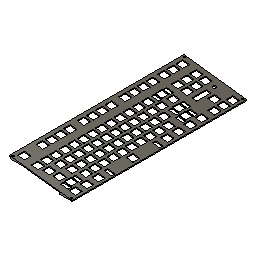
case-top (Autodesk Fusion 360 design; units mm, degrees)
part number: 2025-12-05-19-02-36-904
Autodesk Fusion 360 part; units mm, degrees
(part 1 of 2)
sketch "middle-side-profile" plane through (0, 0, 0) normal (0, 1, 0) x (1, 0, 0)
  line L0 (-127.2538, 3.7478) -> (-128.8538, 3.7478)
  line L1 (-128.8538, -15.8213) -> (-126.4008, -15.5201)
  line L2 (-126.4008, -15.5201) -> (-127.0101, -10.5573)
  line L3 (-128.8538, 3.7478) -> (-128.8538, -15.8213)
  line L4 (-127.0101, -10.5573) -> (-10.504, 3.7478)
  line L5 (-10.504, 3.7478) -> (-56.2538, 3.7478)
  line L6 (0, 0) -> (-128.8538, -15.8213)
  line L7 (-128.8538, 3.7478) -> (0, 3.7478)
  line L8 (0, 3.7478) -> (0, 0)
  line L9 (-24.433, 3.7478) -> (-24.433, -3)
  line L10 (0, 0) -> (-24.433, 0)
  line L11 (-126.3318, -16.082) -> (-126.9165, -11.3197)
  line L12 (-126.7691, -12.5201) -> (-101.9677, -12.5201)
  line L13 (0, 0) -> (0.2437, -1.9851)
  line L14 (-128.8538, -15.8213) -> (-128.6101, -17.8064)
  line L15 (-128.6101, -17.8064) -> (0.2437, -1.9851)
  line L16 (0, 3.7478) -> (1.6, 3.7478)
  line L17 (0.2437, -1.9851) -> (1.6, -1.8186)
  line L18 (1.6, -1.8186) -> (1.6, 3.7478)
  line L19 (0, 0) -> (1.6, 0.1965)
  line L20 (0, 0) -> (1.612, 0) construction
  dimension "d1" = 2
  dimension "d2" = 2
  dimension "d7" = 1.6
  dimension "d8" = 7
  constraint coincident L6.start L8.end
  constraint perpendicular L6 L13
  constraint perpendicular L6 L14
  constraint perpendicular L13 L15
  constraint perpendicular L8 L16
  constraint perpendicular L13 L17
  constraint perpendicular L16 L18
  constraint horizontal L20
  constraint coincident L18 L19.end
  measures "d1" distance of L6.start L13.end
  measures "d2" distance of L1.start L14.end
  measures "d7" distance of L7.end L16.end
  measures "d8" angle of L19 L20
extrude "Extrude1" add sketch "middle-side-profile" along normal blind 362.2 contours L1 L6 L13 L14 L15 | L2 L6 L11 L12 | L13 L17 L18 L19 | L6 L9 L10
sketch "Sketch2" plane through (0, 0, 0) normal (0, 0, -1) x (1, 0, 0)
  line L0 (0, 0) -> (-24.433, 0)
  line L1 (-24.433, 0) -> (-24.433, -362.2)
  line L2 (-24.433, -362.2) -> (0, -362.2)
  line L3 (0, 0) -> (-128.854, 0)
  line L4 (-128.854, 0) -> (-128.854, -362.2)
  line L5 (-128.854, -362.2) -> (0, -362.2)
  line L6 (0, -362.2) -> (0, 0)
  line L7 (0, -362.2) -> (0, 0)
  line L8 (0, -181.1) -> (-128.854, -181.1)
  circle A0 centre (-3.2, -3.2) radius 1.55
  line L9 (1.6, 0) -> (1.6, -362.2)
  circle A1 centre (-124.054, -3.2) radius 1.55
  circle A2 centre (-3.2, -359) radius 1.55
  circle A3 centre (-124.054, -359) radius 1.55
  dimension "d5" = 128.854
  dimension "d6" = 362.2
  dimension "d11" = 181.1
  dimension "d12" = 3.1
  dimension "d13" = 4.8
  dimension "d14" = 3.2
  dimension "d15" = 3.1
  dimension "d16" = 3.2
  dimension "d17" = 4.8
  dimension "d18" = 3.1
  dimension "d19" = 3.2
  dimension "d20" = 4.8
  dimension "d21" = 3.1
  dimension "d22" = 4.8
  dimension "d23" = 3.2
  constraint horizontal L3
  constraint vertical L4
  constraint horizontal L5
  constraint vertical L6
  constraint coincident L0.start L3.start
  constraint coincident L7 L8.start
  constraint coincident L4 L8.end
  constraint perpendicular L4 L8
  measures "d5" distance of L0.start L3.end
  measures "d6" distance of L0.start L2.end
  measures "d11" distance of L5 L8
  measures "d12" diameter of A0
  measures "d13" distance of A0.centre L9
  measures "d14" distance of L3 A0.centre
  measures "d15" diameter of A1
  measures "d16" distance of L3 A1.centre
  measures "d17" distance of L4 A1.centre
  measures "d18" diameter of A2
  measures "d19" distance of L5 A2.centre
  measures "d20" distance of L9 A2.centre
  measures "d21" diameter of A3
  measures "d22" distance of L4 A3.centre
  measures "d23" distance of L5 A3.centre
hole "Hole1" at (-124.054, 359, 0) direction (0, 0, 1) diameter 2.2 depth 15 tip angle 180
hole "Hole2" at (-3.2, 359, 0) direction (0, 0, 1) diameter 2.2 depth 1 tip angle 180
hole "Hole3" at (-3.2, 3.2, 0) direction (0, 0, 1) diameter 2.2 depth 1 tip angle 180
hole "Hole4" at (-124.054, 3.2, 0) direction (0, 0, 1) diameter 2.2 depth 15 tip angle 180
ref_plane "WorkPlane1" through (0, 0, 20) normal (0, 0, 1) x (1, 0, 0)
sketch "Sketch4" plane through (0, 0, 20) normal (0, 0, 1) x (1, 0, 0)
  line L0 (1.6, 0) -> (-128.854, 0)
  line L1 (-128.854, 0) -> (-128.854, -362.2)
  line L2 (-128.854, -362.2) -> (1.6, -362.2)
  line L3 (1.6, -362.2) -> (1.6, 0)
  circle A0 centre (-124.0538, 3.2) radius 2
  line L4 (-128.8538, 0) -> (-128.8538, 362.2)
  circle A1 centre (-124.0538, 359) radius 2
  line L5 (-128.6101, 362.2) -> (1.6, 362.2)
  circle A2 centre (-3.2, 359) radius 2
  line L6 (1.6, 0) -> (1.6, 362.2)
  circle A3 centre (-3.2, 3.2) radius 2
  dimension "d46" = 130.454
  dimension "d47" = 362.2
  dimension "d48" = 4
  dimension "d49" = 4.8
  dimension "d50" = 3.2
  dimension "d51" = 4
  dimension "d52" = 4.8
  dimension "d53" = 3.2
  dimension "d54" = 4
  dimension "d55" = 4.8
  dimension "d56" = 3.2
  dimension "d57" = 4
  dimension "d58" = 3.2
  dimension "d59" = 4.8
  constraint horizontal L0
  constraint vertical L1
  constraint horizontal L2
  constraint vertical L3
  measures "d46" distance of L0.start L0.end
  measures "d47" distance of L0.start L2.end
  measures "d48" diameter of A0
  measures "d49" distance of A0.centre L4
  measures "d50" distance of L0 A0.centre
  measures "d51" diameter of A1
  measures "d52" distance of L4 A1.centre
  measures "d53" distance of A1.centre L5
  measures "d54" diameter of A2
  measures "d55" distance of A2.centre L6
  measures "d56" distance of L5 A2.centre
  measures "d57" diameter of A3
  measures "d58" distance of L0 A3.centre
  measures "d59" distance of L6 A3.centre
hole "Hole6" at (-124.0538, 3.2, 20) direction (0, 0, -1) diameter 4 depth 5 tip angle 180
hole "Hole7" at (-3.2, 3.2, 20) direction (0, 0, -1) diameter 4 depth 19 tip angle 180
hole "Hole8" at (-3.2, 359, 20) direction (0, 0, -1) diameter 4 depth 19 tip angle 180
hole "Hole9" at (-124.0538, 359, 20) direction (0, 0, -1) diameter 4 depth 19 tip angle 180
sketch "plate-2025-12-06T02_04_04.924Z" plane through (0.2437, 0, 1.9851) normal (0.121869, 0, 0.992546) x (0.992546, 0, -0.121869)
  line L0 (-122.5865, 10.3145) -> (-122.5865, 23.3145)
  line L1 (-108.5865, 10.3145) -> (-108.5865, 23.3145)
  line L2 (-122.0865, 9.8145) -> (-109.0865, 9.8145)
  line L3 (-122.0865, 23.8145) -> (-109.0865, 23.8145)
  arc A0 (-122.5865, 10.3145) -> (-122.0865, 9.8145) centre (-122.0865, 10.3145) ccw
  arc A1 (-122.0865, 23.8145) -> (-122.5865, 23.3145) centre (-122.0865, 23.3145) ccw
  arc A2 (-109.0865, 9.8145) -> (-108.5865, 10.3145) centre (-109.0865, 10.3145) ccw
  arc A3 (-108.5865, 23.3145) -> (-109.0865, 23.8145) centre (-109.0865, 23.3145) ccw
  line L4 (-122.5865, 48.4145) -> (-122.5865, 61.4145)
  line L5 (-108.5865, 48.4145) -> (-108.5865, 61.4145)
  line L6 (-122.0865, 47.9145) -> (-109.0865, 47.9145)
  line L7 (-122.0865, 61.9145) -> (-109.0865, 61.9145)
  arc A4 (-122.5865, 48.4145) -> (-122.0865, 47.9145) centre (-122.0865, 48.4145) ccw
  arc A5 (-122.0865, 61.9145) -> (-122.5865, 61.4145) centre (-122.0865, 61.4145) ccw
  arc A6 (-109.0865, 47.9145) -> (-108.5865, 48.4145) centre (-109.0865, 48.4145) ccw
  arc A7 (-108.5865, 61.4145) -> (-109.0865, 61.9145) centre (-109.0865, 61.4145) ccw
  line L8 (-122.5865, 67.4645) -> (-122.5865, 80.4645)
  line L9 (-108.5865, 67.4645) -> (-108.5865, 80.4645)
  line L10 (-122.0865, 66.9645) -> (-109.0865, 66.9645)
  line L11 (-122.0865, 80.9645) -> (-109.0865, 80.9645)
  arc A8 (-122.5865, 67.4645) -> (-122.0865, 66.9645) centre (-122.0865, 67.4645) ccw
  arc A9 (-122.0865, 80.9645) -> (-122.5865, 80.4645) centre (-122.0865, 80.4645) ccw
  arc A10 (-109.0865, 66.9645) -> (-108.5865, 67.4645) centre (-109.0865, 67.4645) ccw
  arc A11 (-108.5865, 80.4645) -> (-109.0865, 80.9645) centre (-109.0865, 80.4645) ccw
  line L12 (-122.5865, 86.5145) -> (-122.5865, 99.5145)
  line L13 (-108.5865, 86.5145) -> (-108.5865, 99.5145)
  line L14 (-122.0865, 86.0145) -> (-109.0865, 86.0145)
  line L15 (-122.0865, 100.0145) -> (-109.0865, 100.0145)
  arc A12 (-122.5865, 86.5145) -> (-122.0865, 86.0145) centre (-122.0865, 86.5145) ccw
  arc A13 (-122.0865, 100.0145) -> (-122.5865, 99.5145) centre (-122.0865, 99.5145) ccw
  arc A14 (-109.0865, 86.0145) -> (-108.5865, 86.5145) centre (-109.0865, 86.5145) ccw
  arc A15 (-108.5865, 99.5145) -> (-109.0865, 100.0145) centre (-109.0865, 99.5145) ccw
  line L16 (-122.5865, 105.5645) -> (-122.5865, 118.5645)
  line L17 (-108.5865, 105.5645) -> (-108.5865, 118.5645)
  line L18 (-122.0865, 105.0645) -> (-109.0865, 105.0645)
  line L19 (-122.0865, 119.0645) -> (-109.0865, 119.0645)
  arc A16 (-122.5865, 105.5645) -> (-122.0865, 105.0645) centre (-122.0865, 105.5645) ccw
  arc A17 (-122.0865, 119.0645) -> (-122.5865, 118.5645) centre (-122.0865, 118.5645) ccw
  arc A18 (-109.0865, 105.0645) -> (-108.5865, 105.5645) centre (-109.0865, 105.5645) ccw
  arc A19 (-108.5865, 118.5645) -> (-109.0865, 119.0645) centre (-109.0865, 118.5645) ccw
  line L20 (-122.5865, 134.1395) -> (-122.5865, 147.1395)
  line L21 (-108.5865, 134.1395) -> (-108.5865, 147.1395)
  line L22 (-122.0865, 133.6395) -> (-109.0865, 133.6395)
  line L23 (-122.0865, 147.6395) -> (-109.0865, 147.6395)
  arc A20 (-122.5865, 134.1395) -> (-122.0865, 133.6395) centre (-122.0865, 134.1395) ccw
  arc A21 (-122.0865, 147.6395) -> (-122.5865, 147.1395) centre (-122.0865, 147.1395) ccw
  arc A22 (-109.0865, 133.6395) -> (-108.5865, 134.1395) centre (-109.0865, 134.1395) ccw
  arc A23 (-108.5865, 147.1395) -> (-109.0865, 147.6395) centre (-109.0865, 147.1395) ccw
  line L24 (-122.5865, 153.1895) -> (-122.5865, 166.1895)
  line L25 (-108.5865, 153.1895) -> (-108.5865, 166.1895)
  line L26 (-122.0865, 152.6895) -> (-109.0865, 152.6895)
  line L27 (-122.0865, 166.6895) -> (-109.0865, 166.6895)
  arc A24 (-122.5865, 153.1895) -> (-122.0865, 152.6895) centre (-122.0865, 153.1895) ccw
  arc A25 (-122.0865, 166.6895) -> (-122.5865, 166.1895) centre (-122.0865, 166.1895) ccw
  arc A26 (-109.0865, 152.6895) -> (-108.5865, 153.1895) centre (-109.0865, 153.1895) ccw
  arc A27 (-108.5865, 166.1895) -> (-109.0865, 166.6895) centre (-109.0865, 166.1895) ccw
  line L28 (-122.5865, 172.2395) -> (-122.5865, 185.2395)
  line L29 (-108.5865, 172.2395) -> (-108.5865, 185.2395)
  line L30 (-122.0865, 171.7395) -> (-109.0865, 171.7395)
  line L31 (-122.0865, 185.7395) -> (-109.0865, 185.7395)
  arc A28 (-122.5865, 172.2395) -> (-122.0865, 171.7395) centre (-122.0865, 172.2395) ccw
  arc A29 (-122.0865, 185.7395) -> (-122.5865, 185.2395) centre (-122.0865, 185.2395) ccw
  arc A30 (-109.0865, 171.7395) -> (-108.5865, 172.2395) centre (-109.0865, 172.2395) ccw
  arc A31 (-108.5865, 185.2395) -> (-109.0865, 185.7395) centre (-109.0865, 185.2395) ccw
  line L32 (-122.5865, 191.2895) -> (-122.5865, 204.2895)
  line L33 (-108.5865, 191.2895) -> (-108.5865, 204.2895)
  line L34 (-122.0865, 190.7895) -> (-109.0865, 190.7895)
  line L35 (-122.0865, 204.7895) -> (-109.0865, 204.7895)
  arc A32 (-122.5865, 191.2895) -> (-122.0865, 190.7895) centre (-122.0865, 191.2895) ccw
  arc A33 (-122.0865, 204.7895) -> (-122.5865, 204.2895) centre (-122.0865, 204.2895) ccw
  arc A34 (-109.0865, 190.7895) -> (-108.5865, 191.2895) centre (-109.0865, 191.2895) ccw
  arc A35 (-108.5865, 204.2895) -> (-109.0865, 204.7895) centre (-109.0865, 204.2895) ccw
  line L36 (-122.5865, 219.8645) -> (-122.5865, 232.8645)
  line L37 (-108.5865, 219.8645) -> (-108.5865, 232.8645)
  line L38 (-122.0865, 219.3645) -> (-109.0865, 219.3645)
  line L39 (-122.0865, 233.3645) -> (-109.0865, 233.3645)
  arc A36 (-122.5865, 219.8645) -> (-122.0865, 219.3645) centre (-122.0865, 219.8645) ccw
  arc A37 (-122.0865, 233.3645) -> (-122.5865, 232.8645) centre (-122.0865, 232.8645) ccw
  arc A38 (-109.0865, 219.3645) -> (-108.5865, 219.8645) centre (-109.0865, 219.8645) ccw
  arc A39 (-108.5865, 232.8645) -> (-109.0865, 233.3645) centre (-109.0865, 232.8645) ccw
  line L40 (-122.5865, 238.9145) -> (-122.5865, 251.9145)
  line L41 (-108.5865, 238.9145) -> (-108.5865, 251.9145)
  line L42 (-122.0865, 238.4145) -> (-109.0865, 238.4145)
  line L43 (-122.0865, 252.4145) -> (-109.0865, 252.4145)
  arc A40 (-122.5865, 238.9145) -> (-122.0865, 238.4145) centre (-122.0865, 238.9145) ccw
  arc A41 (-122.0865, 252.4145) -> (-122.5865, 251.9145) centre (-122.0865, 251.9145) ccw
  arc A42 (-109.0865, 238.4145) -> (-108.5865, 238.9145) centre (-109.0865, 238.9145) ccw
  arc A43 (-108.5865, 251.9145) -> (-109.0865, 252.4145) centre (-109.0865, 251.9145) ccw
  line L44 (-122.5865, 257.9645) -> (-122.5865, 270.9645)
  line L45 (-108.5865, 257.9645) -> (-108.5865, 270.9645)
  line L46 (-122.0865, 257.4645) -> (-109.0865, 257.4645)
  line L47 (-122.0865, 271.4645) -> (-109.0865, 271.4645)
  arc A44 (-122.5865, 257.9645) -> (-122.0865, 257.4645) centre (-122.0865, 257.9645) ccw
  arc A45 (-122.0865, 271.4645) -> (-122.5865, 270.9645) centre (-122.0865, 270.9645) ccw
  arc A46 (-109.0865, 257.4645) -> (-108.5865, 257.9645) centre (-109.0865, 257.9645) ccw
  arc A47 (-108.5865, 270.9645) -> (-109.0865, 271.4645) centre (-109.0865, 270.9645) ccw
  line L48 (-122.5865, 277.0145) -> (-122.5865, 290.0145)
  line L49 (-108.5865, 277.0145) -> (-108.5865, 290.0145)
  line L50 (-122.0865, 276.5145) -> (-109.0865, 276.5145)
  line L51 (-122.0865, 290.5145) -> (-109.0865, 290.5145)
  arc A48 (-122.5865, 277.0145) -> (-122.0865, 276.5145) centre (-122.0865, 277.0145) ccw
  arc A49 (-122.0865, 290.5145) -> (-122.5865, 290.0145) centre (-122.0865, 290.0145) ccw
  arc A50 (-109.0865, 276.5145) -> (-108.5865, 277.0145) centre (-109.0865, 277.0145) ccw
  arc A51 (-108.5865, 290.0145) -> (-109.0865, 290.5145) centre (-109.0865, 290.0145) ccw
  line L52 (-122.5865, 300.827) -> (-122.5865, 313.827)
  line L53 (-108.5865, 300.827) -> (-108.5865, 313.827)
  line L54 (-122.0865, 300.327) -> (-109.0865, 300.327)
  line L55 (-122.0865, 314.327) -> (-109.0865, 314.327)
  arc A52 (-122.5865, 300.827) -> (-122.0865, 300.327) centre (-122.0865, 300.827) ccw
  arc A53 (-122.0865, 314.327) -> (-122.5865, 313.827) centre (-122.0865, 313.827) ccw
  arc A54 (-109.0865, 300.327) -> (-108.5865, 300.827) centre (-109.0865, 300.827) ccw
  arc A55 (-108.5865, 313.827) -> (-109.0865, 314.327) centre (-109.0865, 313.827) ccw
  line L56 (-122.5865, 319.877) -> (-122.5865, 332.877)
  line L57 (-108.5865, 319.877) -> (-108.5865, 332.877)
  line L58 (-122.0865, 319.377) -> (-109.0865, 319.377)
  line L59 (-122.0865, 333.377) -> (-109.0865, 333.377)
  arc A56 (-122.5865, 319.877) -> (-122.0865, 319.377) centre (-122.0865, 319.877) ccw
  arc A57 (-122.0865, 333.377) -> (-122.5865, 332.877) centre (-122.0865, 332.877) ccw
  arc A58 (-109.0865, 319.377) -> (-108.5865, 319.877) centre (-109.0865, 319.877) ccw
  arc A59 (-108.5865, 332.877) -> (-109.0865, 333.377) centre (-109.0865, 332.877) ccw
  line L60 (-122.5865, 338.927) -> (-122.5865, 351.927)
  line L61 (-108.5865, 338.927) -> (-108.5865, 351.927)
  line L62 (-122.0865, 338.427) -> (-109.0865, 338.427)
  line L63 (-122.0865, 352.427) -> (-109.0865, 352.427)
  arc A60 (-122.5865, 338.927) -> (-122.0865, 338.427) centre (-122.0865, 338.927) ccw
  arc A61 (-122.0865, 352.427) -> (-122.5865, 351.927) centre (-122.0865, 351.927) ccw
  arc A62 (-109.0865, 338.427) -> (-108.5865, 338.927) centre (-109.0865, 338.927) ccw
  arc A63 (-108.5865, 351.927) -> (-109.0865, 352.427) centre (-109.0865, 351.927) ccw
  line L64 (-94.0115, 10.3145) -> (-94.0115, 23.3145)
  line L65 (-80.0115, 10.3145) -> (-80.0115, 23.3145)
  line L66 (-93.5115, 9.8145) -> (-80.5115, 9.8145)
  line L67 (-93.5115, 23.8145) -> (-80.5115, 23.8145)
  arc A64 (-94.0115, 10.3145) -> (-93.5115, 9.8145) centre (-93.5115, 10.3145) ccw
  arc A65 (-93.5115, 23.8145) -> (-94.0115, 23.3145) centre (-93.5115, 23.3145) ccw
  arc A66 (-80.5115, 9.8145) -> (-80.0115, 10.3145) centre (-80.5115, 10.3145) ccw
  arc A67 (-80.0115, 23.3145) -> (-80.5115, 23.8145) centre (-80.5115, 23.3145) ccw
  line L68 (-94.0115, 29.3645) -> (-94.0115, 42.3645)
  line L69 (-80.0115, 29.3645) -> (-80.0115, 42.3645)
  line L70 (-93.5115, 28.8645) -> (-80.5115, 28.8645)
  line L71 (-93.5115, 42.8645) -> (-80.5115, 42.8645)
  arc A68 (-94.0115, 29.3645) -> (-93.5115, 28.8645) centre (-93.5115, 29.3645) ccw
  arc A69 (-93.5115, 42.8645) -> (-94.0115, 42.3645) centre (-93.5115, 42.3645) ccw
  arc A70 (-80.5115, 28.8645) -> (-80.0115, 29.3645) centre (-80.5115, 29.3645) ccw
  arc A71 (-80.0115, 42.3645) -> (-80.5115, 42.8645) centre (-80.5115, 42.3645) ccw
  line L72 (-94.0115, 48.4145) -> (-94.0115, 61.4145)
  line L73 (-80.0115, 48.4145) -> (-80.0115, 61.4145)
  line L74 (-93.5115, 47.9145) -> (-80.5115, 47.9145)
  line L75 (-93.5115, 61.9145) -> (-80.5115, 61.9145)
  arc A72 (-94.0115, 48.4145) -> (-93.5115, 47.9145) centre (-93.5115, 48.4145) ccw
  arc A73 (-93.5115, 61.9145) -> (-94.0115, 61.4145) centre (-93.5115, 61.4145) ccw
  arc A74 (-80.5115, 47.9145) -> (-80.0115, 48.4145) centre (-80.5115, 48.4145) ccw
  arc A75 (-80.0115, 61.4145) -> (-80.5115, 61.9145) centre (-80.5115, 61.4145) ccw
  line L76 (-94.0115, 67.4645) -> (-94.0115, 80.4645)
  line L77 (-80.0115, 67.4645) -> (-80.0115, 80.4645)
  line L78 (-93.5115, 66.9645) -> (-80.5115, 66.9645)
  line L79 (-93.5115, 80.9645) -> (-80.5115, 80.9645)
  arc A76 (-94.0115, 67.4645) -> (-93.5115, 66.9645) centre (-93.5115, 67.4645) ccw
  arc A77 (-93.5115, 80.9645) -> (-94.0115, 80.4645) centre (-93.5115, 80.4645) ccw
  arc A78 (-80.5115, 66.9645) -> (-80.0115, 67.4645) centre (-80.5115, 67.4645) ccw
  arc A79 (-80.0115, 80.4645) -> (-80.5115, 80.9645) centre (-80.5115, 80.4645) ccw
  line L80 (-94.0115, 86.5145) -> (-94.0115, 99.5145)
  line L81 (-80.0115, 86.5145) -> (-80.0115, 99.5145)
  line L82 (-93.5115, 86.0145) -> (-80.5115, 86.0145)
  line L83 (-93.5115, 100.0145) -> (-80.5115, 100.0145)
  arc A80 (-94.0115, 86.5145) -> (-93.5115, 86.0145) centre (-93.5115, 86.5145) ccw
  arc A81 (-93.5115, 100.0145) -> (-94.0115, 99.5145) centre (-93.5115, 99.5145) ccw
  arc A82 (-80.5115, 86.0145) -> (-80.0115, 86.5145) centre (-80.5115, 86.5145) ccw
  arc A83 (-80.0115, 99.5145) -> (-80.5115, 100.0145) centre (-80.5115, 99.5145) ccw
  line L84 (-94.0115, 105.5645) -> (-94.0115, 118.5645)
  line L85 (-80.0115, 105.5645) -> (-80.0115, 118.5645)
  line L86 (-93.5115, 105.0645) -> (-80.5115, 105.0645)
  line L87 (-93.5115, 119.0645) -> (-80.5115, 119.0645)
  arc A84 (-94.0115, 105.5645) -> (-93.5115, 105.0645) centre (-93.5115, 105.5645) ccw
  arc A85 (-93.5115, 119.0645) -> (-94.0115, 118.5645) centre (-93.5115, 118.5645) ccw
  arc A86 (-80.5115, 105.0645) -> (-80.0115, 105.5645) centre (-80.5115, 105.5645) ccw
  arc A87 (-80.0115, 118.5645) -> (-80.5115, 119.0645) centre (-80.5115, 118.5645) ccw
  line L88 (-94.0115, 124.6145) -> (-94.0115, 137.6145)
  line L89 (-80.0115, 124.6145) -> (-80.0115, 137.6145)
  line L90 (-93.5115, 124.1145) -> (-80.5115, 124.1145)
  line L91 (-93.5115, 138.1145) -> (-80.5115, 138.1145)
  arc A88 (-94.0115, 124.6145) -> (-93.5115, 124.1145) centre (-93.5115, 124.6145) ccw
  arc A89 (-93.5115, 138.1145) -> (-94.0115, 137.6145) centre (-93.5115, 137.6145) ccw
  arc A90 (-80.5115, 124.1145) -> (-80.0115, 124.6145) centre (-80.5115, 124.6145) ccw
  arc A91 (-80.0115, 137.6145) -> (-80.5115, 138.1145) centre (-80.5115, 137.6145) ccw
  line L92 (-94.0115, 143.6645) -> (-94.0115, 156.6645)
  line L93 (-80.0115, 143.6645) -> (-80.0115, 156.6645)
  line L94 (-93.5115, 143.1645) -> (-80.5115, 143.1645)
  line L95 (-93.5115, 157.1645) -> (-80.5115, 157.1645)
  arc A92 (-94.0115, 143.6645) -> (-93.5115, 143.1645) centre (-93.5115, 143.6645) ccw
  arc A93 (-93.5115, 157.1645) -> (-94.0115, 156.6645) centre (-93.5115, 156.6645) ccw
  arc A94 (-80.5115, 143.1645) -> (-80.0115, 143.6645) centre (-80.5115, 143.6645) ccw
  arc A95 (-80.0115, 156.6645) -> (-80.5115, 157.1645) centre (-80.5115, 156.6645) ccw
  line L96 (-94.0115, 162.7145) -> (-94.0115, 175.7145)
  line L97 (-80.0115, 162.7145) -> (-80.0115, 175.7145)
  line L98 (-93.5115, 162.2145) -> (-80.5115, 162.2145)
  line L99 (-93.5115, 176.2145) -> (-80.5115, 176.2145)
  arc A96 (-94.0115, 162.7145) -> (-93.5115, 162.2145) centre (-93.5115, 162.7145) ccw
  arc A97 (-93.5115, 176.2145) -> (-94.0115, 175.7145) centre (-93.5115, 175.7145) ccw
  arc A98 (-80.5115, 162.2145) -> (-80.0115, 162.7145) centre (-80.5115, 162.7145) ccw
  arc A99 (-80.0115, 175.7145) -> (-80.5115, 176.2145) centre (-80.5115, 175.7145) ccw
  line L100 (-94.0115, 181.7645) -> (-94.0115, 194.7645)
  line L101 (-80.0115, 181.7645) -> (-80.0115, 194.7645)
  line L102 (-93.5115, 181.2645) -> (-80.5115, 181.2645)
  line L103 (-93.5115, 195.2645) -> (-80.5115, 195.2645)
  arc A100 (-94.0115, 181.7645) -> (-93.5115, 181.2645) centre (-93.5115, 181.7645) ccw
  arc A101 (-93.5115, 195.2645) -> (-94.0115, 194.7645) centre (-93.5115, 194.7645) ccw
  arc A102 (-80.5115, 181.2645) -> (-80.0115, 181.7645) centre (-80.5115, 181.7645) ccw
  arc A103 (-80.0115, 194.7645) -> (-80.5115, 195.2645) centre (-80.5115, 194.7645) ccw
  line L104 (-94.0115, 200.8145) -> (-94.0115, 213.8145)
  line L105 (-80.0115, 200.8145) -> (-80.0115, 213.8145)
  line L106 (-93.5115, 200.3145) -> (-80.5115, 200.3145)
  line L107 (-93.5115, 214.3145) -> (-80.5115, 214.3145)
  arc A104 (-94.0115, 200.8145) -> (-93.5115, 200.3145) centre (-93.5115, 200.8145) ccw
  arc A105 (-93.5115, 214.3145) -> (-94.0115, 213.8145) centre (-93.5115, 213.8145) ccw
  arc A106 (-80.5115, 200.3145) -> (-80.0115, 200.8145) centre (-80.5115, 200.8145) ccw
  arc A107 (-80.0115, 213.8145) -> (-80.5115, 214.3145) centre (-80.5115, 213.8145) ccw
  line L108 (-94.0115, 219.8645) -> (-94.0115, 232.8645)
  line L109 (-80.0115, 219.8645) -> (-80.0115, 232.8645)
  line L110 (-93.5115, 219.3645) -> (-80.5115, 219.3645)
  line L111 (-93.5115, 233.3645) -> (-80.5115, 233.3645)
  arc A108 (-94.0115, 219.8645) -> (-93.5115, 219.3645) centre (-93.5115, 219.8645) ccw
  arc A109 (-93.5115, 233.3645) -> (-94.0115, 232.8645) centre (-93.5115, 232.8645) ccw
  arc A110 (-80.5115, 219.3645) -> (-80.0115, 219.8645) centre (-80.5115, 219.8645) ccw
  arc A111 (-80.0115, 232.8645) -> (-80.5115, 233.3645) centre (-80.5115, 232.8645) ccw
  line L112 (-94.0115, 238.9145) -> (-94.0115, 251.9145)
  line L113 (-80.0115, 238.9145) -> (-80.0115, 251.9145)
  line L114 (-93.5115, 238.4145) -> (-80.5115, 238.4145)
  line L115 (-93.5115, 252.4145) -> (-80.5115, 252.4145)
  arc A112 (-94.0115, 238.9145) -> (-93.5115, 238.4145) centre (-93.5115, 238.9145) ccw
  arc A113 (-93.5115, 252.4145) -> (-94.0115, 251.9145) centre (-93.5115, 251.9145) ccw
  arc A114 (-80.5115, 238.4145) -> (-80.0115, 238.9145) centre (-80.5115, 238.9145) ccw
  arc A115 (-80.0115, 251.9145) -> (-80.5115, 252.4145) centre (-80.5115, 251.9145) ccw
  line L116 (-94.0115, 267.4895) -> (-94.0115, 280.4895)
  line L117 (-80.0115, 267.4895) -> (-80.0115, 280.4895)
  line L118 (-93.5115, 266.9895) -> (-80.5115, 266.9895)
  line L119 (-93.5115, 280.9895) -> (-80.5115, 280.9895)
  arc A116 (-94.0115, 267.4895) -> (-93.5115, 266.9895) centre (-93.5115, 267.4895) ccw
  arc A117 (-93.5115, 280.9895) -> (-94.0115, 280.4895) centre (-93.5115, 280.4895) ccw
  arc A118 (-80.5115, 266.9895) -> (-80.0115, 267.4895) centre (-80.5115, 267.4895) ccw
  arc A119 (-80.0115, 280.4895) -> (-80.5115, 280.9895) centre (-80.5115, 280.4895) ccw
  line L120 (-93.0115, 259.0515) -> (-93.0115, 265.0515)
  line L121 (-78.0115, 259.0515) -> (-78.0115, 265.0515)
  line L122 (-92.5115, 258.5515) -> (-78.5115, 258.5515)
  line L123 (-92.5115, 265.5515) -> (-78.5115, 265.5515)
  arc A120 (-93.0115, 259.0515) -> (-92.5115, 258.5515) centre (-92.5115, 259.0515) ccw
  arc A121 (-92.5115, 265.5515) -> (-93.0115, 265.0515) centre (-92.5115, 265.0515) ccw
  arc A122 (-78.5115, 258.5515) -> (-78.0115, 259.0515) centre (-78.5115, 259.0515) ccw
  arc A123 (-78.0115, 265.0515) -> (-78.5115, 265.5515) centre (-78.5115, 265.0515) ccw
  line L124 (-93.0115, 282.9275) -> (-93.0115, 288.9275)
  line L125 (-78.0115, 282.9275) -> (-78.0115, 288.9275)
  line L126 (-92.5115, 282.4275) -> (-78.5115, 282.4275)
  line L127 (-92.5115, 289.4275) -> (-78.5115, 289.4275)
  arc A124 (-93.0115, 282.9275) -> (-92.5115, 282.4275) centre (-92.5115, 282.9275) ccw
  arc A125 (-92.5115, 289.4275) -> (-93.0115, 288.9275) centre (-92.5115, 288.9275) ccw
  arc A126 (-78.5115, 282.4275) -> (-78.0115, 282.9275) centre (-78.5115, 282.9275) ccw
  arc A127 (-78.0115, 288.9275) -> (-78.5115, 289.4275) centre (-78.5115, 288.9275) ccw
  line L128 (-94.0115, 300.827) -> (-94.0115, 313.827)
  line L129 (-80.0115, 300.827) -> (-80.0115, 313.827)
  line L130 (-93.5115, 300.327) -> (-80.5115, 300.327)
  line L131 (-93.5115, 314.327) -> (-80.5115, 314.327)
  arc A128 (-94.0115, 300.827) -> (-93.5115, 300.327) centre (-93.5115, 300.827) ccw
  arc A129 (-93.5115, 314.327) -> (-94.0115, 313.827) centre (-93.5115, 313.827) ccw
  arc A130 (-80.5115, 300.327) -> (-80.0115, 300.827) centre (-80.5115, 300.827) ccw
  arc A131 (-80.0115, 313.827) -> (-80.5115, 314.327) centre (-80.5115, 313.827) ccw
  line L132 (-94.0115, 319.877) -> (-94.0115, 332.877)
  line L133 (-80.0115, 319.877) -> (-80.0115, 332.877)
  line L134 (-93.5115, 319.377) -> (-80.5115, 319.377)
  line L135 (-93.5115, 333.377) -> (-80.5115, 333.377)
  arc A132 (-94.0115, 319.877) -> (-93.5115, 319.377) centre (-93.5115, 319.877) ccw
  arc A133 (-93.5115, 333.377) -> (-94.0115, 332.877) centre (-93.5115, 332.877) ccw
  arc A134 (-80.5115, 319.377) -> (-80.0115, 319.877) centre (-80.5115, 319.877) ccw
  arc A135 (-80.0115, 332.877) -> (-80.5115, 333.377) centre (-80.5115, 332.877) ccw
  line L136 (-94.0115, 338.927) -> (-94.0115, 351.927)
  line L137 (-80.0115, 338.927) -> (-80.0115, 351.927)
  line L138 (-93.5115, 338.427) -> (-80.5115, 338.427)
  line L139 (-93.5115, 352.427) -> (-80.5115, 352.427)
  arc A136 (-94.0115, 338.927) -> (-93.5115, 338.427) centre (-93.5115, 338.927) ccw
  arc A137 (-93.5115, 352.427) -> (-94.0115, 351.927) centre (-93.5115, 351.927) ccw
  arc A138 (-80.5115, 338.427) -> (-80.0115, 338.927) centre (-80.5115, 338.927) ccw
  arc A139 (-80.0115, 351.927) -> (-80.5115, 352.427) centre (-80.5115, 351.927) ccw
  line L140 (-74.9615, 15.077) -> (-74.9615, 28.077)
  line L141 (-60.9615, 15.077) -> (-60.9615, 28.077)
  line L142 (-74.4615, 14.577) -> (-61.4615, 14.577)
  line L143 (-74.4615, 28.577) -> (-61.4615, 28.577)
  arc A140 (-74.9615, 15.077) -> (-74.4615, 14.577) centre (-74.4615, 15.077) ccw
  arc A141 (-74.4615, 28.577) -> (-74.9615, 28.077) centre (-74.4615, 28.077) ccw
  arc A142 (-61.4615, 14.577) -> (-60.9615, 15.077) centre (-61.4615, 15.077) ccw
  arc A143 (-60.9615, 28.077) -> (-61.4615, 28.577) centre (-61.4615, 28.077) ccw
  line L144 (-74.9615, 38.8895) -> (-74.9615, 51.8895)
  line L145 (-60.9615, 38.8895) -> (-60.9615, 51.8895)
  line L146 (-74.4615, 38.3895) -> (-61.4615, 38.3895)
  line L147 (-74.4615, 52.3895) -> (-61.4615, 52.3895)
  arc A144 (-74.9615, 38.8895) -> (-74.4615, 38.3895) centre (-74.4615, 38.8895) ccw
  arc A145 (-74.4615, 52.3895) -> (-74.9615, 51.8895) centre (-74.4615, 51.8895) ccw
  arc A146 (-61.4615, 38.3895) -> (-60.9615, 38.8895) centre (-61.4615, 38.8895) ccw
  arc A147 (-60.9615, 51.8895) -> (-61.4615, 52.3895) centre (-61.4615, 51.8895) ccw
  line L148 (-74.9615, 57.9395) -> (-74.9615, 70.9395)
  line L149 (-60.9615, 57.9395) -> (-60.9615, 70.9395)
  line L150 (-74.4615, 57.4395) -> (-61.4615, 57.4395)
  line L151 (-74.4615, 71.4395) -> (-61.4615, 71.4395)
  arc A148 (-74.9615, 57.9395) -> (-74.4615, 57.4395) centre (-74.4615, 57.9395) ccw
  arc A149 (-74.4615, 71.4395) -> (-74.9615, 70.9395) centre (-74.4615, 70.9395) ccw
  arc A150 (-61.4615, 57.4395) -> (-60.9615, 57.9395) centre (-61.4615, 57.9395) ccw
  arc A151 (-60.9615, 70.9395) -> (-61.4615, 71.4395) centre (-61.4615, 70.9395) ccw
  line L152 (-74.9615, 76.9895) -> (-74.9615, 89.9895)
  line L153 (-60.9615, 76.9895) -> (-60.9615, 89.9895)
  line L154 (-74.4615, 76.4895) -> (-61.4615, 76.4895)
  line L155 (-74.4615, 90.4895) -> (-61.4615, 90.4895)
  arc A152 (-74.9615, 76.9895) -> (-74.4615, 76.4895) centre (-74.4615, 76.9895) ccw
  arc A153 (-74.4615, 90.4895) -> (-74.9615, 89.9895) centre (-74.4615, 89.9895) ccw
  arc A154 (-61.4615, 76.4895) -> (-60.9615, 76.9895) centre (-61.4615, 76.9895) ccw
  arc A155 (-60.9615, 89.9895) -> (-61.4615, 90.4895) centre (-61.4615, 89.9895) ccw
  line L156 (-74.9615, 96.0395) -> (-74.9615, 109.0395)
  line L157 (-60.9615, 96.0395) -> (-60.9615, 109.0395)
  line L158 (-74.4615, 95.5395) -> (-61.4615, 95.5395)
  line L159 (-74.4615, 109.5395) -> (-61.4615, 109.5395)
  arc A156 (-74.9615, 96.0395) -> (-74.4615, 95.5395) centre (-74.4615, 96.0395) ccw
  arc A157 (-74.4615, 109.5395) -> (-74.9615, 109.0395) centre (-74.4615, 109.0395) ccw
  arc A158 (-61.4615, 95.5395) -> (-60.9615, 96.0395) centre (-61.4615, 96.0395) ccw
  arc A159 (-60.9615, 109.0395) -> (-61.4615, 109.5395) centre (-61.4615, 109.0395) ccw
  line L160 (-74.9615, 115.0895) -> (-74.9615, 128.0895)
  line L161 (-60.9615, 115.0895) -> (-60.9615, 128.0895)
  line L162 (-74.4615, 114.5895) -> (-61.4615, 114.5895)
  line L163 (-74.4615, 128.5895) -> (-61.4615, 128.5895)
  arc A160 (-74.9615, 115.0895) -> (-74.4615, 114.5895) centre (-74.4615, 115.0895) ccw
  arc A161 (-74.4615, 128.5895) -> (-74.9615, 128.0895) centre (-74.4615, 128.0895) ccw
  arc A162 (-61.4615, 114.5895) -> (-60.9615, 115.0895) centre (-61.4615, 115.0895) ccw
  arc A163 (-60.9615, 128.0895) -> (-61.4615, 128.5895) centre (-61.4615, 128.0895) ccw
  line L164 (-74.9615, 134.1395) -> (-74.9615, 147.1395)
  line L165 (-60.9615, 134.1395) -> (-60.9615, 147.1395)
  line L166 (-74.4615, 133.6395) -> (-61.4615, 133.6395)
  line L167 (-74.4615, 147.6395) -> (-61.4615, 147.6395)
  arc A164 (-74.9615, 134.1395) -> (-74.4615, 133.6395) centre (-74.4615, 134.1395) ccw
  arc A165 (-74.4615, 147.6395) -> (-74.9615, 147.1395) centre (-74.4615, 147.1395) ccw
  arc A166 (-61.4615, 133.6395) -> (-60.9615, 134.1395) centre (-61.4615, 134.1395) ccw
  arc A167 (-60.9615, 147.1395) -> (-61.4615, 147.6395) centre (-61.4615, 147.1395) ccw
  line L168 (-74.9615, 153.1895) -> (-74.9615, 166.1895)
  line L169 (-60.9615, 153.1895) -> (-60.9615, 166.1895)
  line L170 (-74.4615, 152.6895) -> (-61.4615, 152.6895)
  line L171 (-74.4615, 166.6895) -> (-61.4615, 166.6895)
  arc A168 (-74.9615, 153.1895) -> (-74.4615, 152.6895) centre (-74.4615, 153.1895) ccw
  arc A169 (-74.4615, 166.6895) -> (-74.9615, 166.1895) centre (-74.4615, 166.1895) ccw
  arc A170 (-61.4615, 152.6895) -> (-60.9615, 153.1895) centre (-61.4615, 153.1895) ccw
  arc A171 (-60.9615, 166.1895) -> (-61.4615, 166.6895) centre (-61.4615, 166.1895) ccw
  line L172 (-74.9615, 172.2395) -> (-74.9615, 185.2395)
  line L173 (-60.9615, 172.2395) -> (-60.9615, 185.2395)
  line L174 (-74.4615, 171.7395) -> (-61.4615, 171.7395)
  line L175 (-74.4615, 185.7395) -> (-61.4615, 185.7395)
  arc A172 (-74.9615, 172.2395) -> (-74.4615, 171.7395) centre (-74.4615, 172.2395) ccw
  arc A173 (-74.4615, 185.7395) -> (-74.9615, 185.2395) centre (-74.4615, 185.2395) ccw
  arc A174 (-61.4615, 171.7395) -> (-60.9615, 172.2395) centre (-61.4615, 172.2395) ccw
  arc A175 (-60.9615, 185.2395) -> (-61.4615, 185.7395) centre (-61.4615, 185.2395) ccw
  line L176 (-74.9615, 191.2895) -> (-74.9615, 204.2895)
  line L177 (-60.9615, 191.2895) -> (-60.9615, 204.2895)
  line L178 (-74.4615, 190.7895) -> (-61.4615, 190.7895)
  line L179 (-74.4615, 204.7895) -> (-61.4615, 204.7895)
  arc A176 (-74.9615, 191.2895) -> (-74.4615, 190.7895) centre (-74.4615, 191.2895) ccw
  arc A177 (-74.4615, 204.7895) -> (-74.9615, 204.2895) centre (-74.4615, 204.2895) ccw
  arc A178 (-61.4615, 190.7895) -> (-60.9615, 191.2895) centre (-61.4615, 191.2895) ccw
  arc A179 (-60.9615, 204.2895) -> (-61.4615, 204.7895) centre (-61.4615, 204.2895) ccw
  line L180 (-74.9615, 210.3395) -> (-74.9615, 223.3395)
  line L181 (-60.9615, 210.3395) -> (-60.9615, 223.3395)
  line L182 (-74.4615, 209.8395) -> (-61.4615, 209.8395)
  line L183 (-74.4615, 223.8395) -> (-61.4615, 223.8395)
  arc A180 (-74.9615, 210.3395) -> (-74.4615, 209.8395) centre (-74.4615, 210.3395) ccw
  arc A181 (-74.4615, 223.8395) -> (-74.9615, 223.3395) centre (-74.4615, 223.3395) ccw
  arc A182 (-61.4615, 209.8395) -> (-60.9615, 210.3395) centre (-61.4615, 210.3395) ccw
  arc A183 (-60.9615, 223.3395) -> (-61.4615, 223.8395) centre (-61.4615, 223.3395) ccw
  line L184 (-74.9615, 229.3895) -> (-74.9615, 242.3895)
  line L185 (-60.9615, 229.3895) -> (-60.9615, 242.3895)
  line L186 (-74.4615, 228.8895) -> (-61.4615, 228.8895)
  line L187 (-74.4615, 242.8895) -> (-61.4615, 242.8895)
  arc A184 (-74.9615, 229.3895) -> (-74.4615, 228.8895) centre (-74.4615, 229.3895) ccw
  arc A185 (-74.4615, 242.8895) -> (-74.9615, 242.3895) centre (-74.4615, 242.3895) ccw
  arc A186 (-61.4615, 228.8895) -> (-60.9615, 229.3895) centre (-61.4615, 229.3895) ccw
  arc A187 (-60.9615, 242.3895) -> (-61.4615, 242.8895) centre (-61.4615, 242.3895) ccw
  line L188 (-74.9615, 248.4395) -> (-74.9615, 261.4395)
  line L189 (-60.9615, 248.4395) -> (-60.9615, 261.4395)
  line L190 (-74.4615, 247.9395) -> (-61.4615, 247.9395)
  line L191 (-74.4615, 261.9395) -> (-61.4615, 261.9395)
  arc A188 (-74.9615, 248.4395) -> (-74.4615, 247.9395) centre (-74.4615, 248.4395) ccw
  arc A189 (-74.4615, 261.9395) -> (-74.9615, 261.4395) centre (-74.4615, 261.4395) ccw
  arc A190 (-61.4615, 247.9395) -> (-60.9615, 248.4395) centre (-61.4615, 248.4395) ccw
  arc A191 (-60.9615, 261.4395) -> (-61.4615, 261.9395) centre (-61.4615, 261.4395) ccw
  line L192 (-74.9615, 272.252) -> (-74.9615, 285.252)
  line L193 (-60.9615, 272.252) -> (-60.9615, 285.252)
  line L194 (-74.4615, 271.752) -> (-61.4615, 271.752)
  line L195 (-74.4615, 285.752) -> (-61.4615, 285.752)
  arc A192 (-74.9615, 272.252) -> (-74.4615, 271.752) centre (-74.4615, 272.252) ccw
  arc A193 (-74.4615, 285.752) -> (-74.9615, 285.252) centre (-74.4615, 285.252) ccw
  arc A194 (-61.4615, 271.752) -> (-60.9615, 272.252) centre (-61.4615, 272.252) ccw
  arc A195 (-60.9615, 285.252) -> (-61.4615, 285.752) centre (-61.4615, 285.252) ccw
  line L196 (-74.9615, 300.827) -> (-74.9615, 313.827)
  line L197 (-60.9615, 300.827) -> (-60.9615, 313.827)
  line L198 (-74.4615, 300.327) -> (-61.4615, 300.327)
  line L199 (-74.4615, 314.327) -> (-61.4615, 314.327)
  arc A196 (-74.9615, 300.827) -> (-74.4615, 300.327) centre (-74.4615, 300.827) ccw
  arc A197 (-74.4615, 314.327) -> (-74.9615, 313.827) centre (-74.4615, 313.827) ccw
  arc A198 (-61.4615, 300.327) -> (-60.9615, 300.827) centre (-61.4615, 300.827) ccw
  arc A199 (-60.9615, 313.827) -> (-61.4615, 314.327) centre (-61.4615, 313.827) ccw
  line L200 (-74.9615, 319.877) -> (-74.9615, 332.877)
  line L201 (-60.9615, 319.877) -> (-60.9615, 332.877)
  line L202 (-74.4615, 319.377) -> (-61.4615, 319.377)
  line L203 (-74.4615, 333.377) -> (-61.4615, 333.377)
  arc A200 (-74.9615, 319.877) -> (-74.4615, 319.377) centre (-74.4615, 319.877) ccw
  arc A201 (-74.4615, 333.377) -> (-74.9615, 332.877) centre (-74.4615, 332.877) ccw
  arc A202 (-61.4615, 319.377) -> (-60.9615, 319.877) centre (-61.4615, 319.877) ccw
  arc A203 (-60.9615, 332.877) -> (-61.4615, 333.377) centre (-61.4615, 332.877) ccw
  line L204 (-74.9615, 338.927) -> (-74.9615, 351.927)
  line L205 (-60.9615, 338.927) -> (-60.9615, 351.927)
  line L206 (-74.4615, 338.427) -> (-61.4615, 338.427)
  line L207 (-74.4615, 352.427) -> (-61.4615, 352.427)
  arc A204 (-74.9615, 338.927) -> (-74.4615, 338.427) centre (-74.4615, 338.927) ccw
  arc A205 (-74.4615, 352.427) -> (-74.9615, 351.927) centre (-74.4615, 351.927) ccw
  arc A206 (-61.4615, 338.427) -> (-60.9615, 338.927) centre (-61.4615, 338.927) ccw
  arc A207 (-60.9615, 351.927) -> (-61.4615, 352.427) centre (-61.4615, 351.927) ccw
  line L208 (-55.9115, 17.4582) -> (-55.9115, 30.4582)
  line L209 (-41.9115, 17.4582) -> (-41.9115, 30.4582)
  line L210 (-55.4115, 16.9582) -> (-42.4115, 16.9582)
  line L211 (-55.4115, 30.9582) -> (-42.4115, 30.9582)
  arc A208 (-55.9115, 17.4582) -> (-55.4115, 16.9582) centre (-55.4115, 17.4582) ccw
  arc A209 (-55.4115, 30.9582) -> (-55.9115, 30.4582) centre (-55.4115, 30.4582) ccw
  arc A210 (-42.4115, 16.9582) -> (-41.9115, 17.4582) centre (-42.4115, 17.4582) ccw
  arc A211 (-41.9115, 30.4582) -> (-42.4115, 30.9582) centre (-42.4115, 30.4582) ccw
  line L212 (-55.9115, 43.652) -> (-55.9115, 56.652)
  line L213 (-41.9115, 43.652) -> (-41.9115, 56.652)
  line L214 (-55.4115, 43.152) -> (-42.4115, 43.152)
  line L215 (-55.4115, 57.152) -> (-42.4115, 57.152)
  arc A212 (-55.9115, 43.652) -> (-55.4115, 43.152) centre (-55.4115, 43.652) ccw
  arc A213 (-55.4115, 57.152) -> (-55.9115, 56.652) centre (-55.4115, 56.652) ccw
  arc A214 (-42.4115, 43.152) -> (-41.9115, 43.652) centre (-42.4115, 43.652) ccw
  arc A215 (-41.9115, 56.652) -> (-42.4115, 57.152) centre (-42.4115, 56.652) ccw
  line L216 (-55.9115, 62.702) -> (-55.9115, 75.702)
  line L217 (-41.9115, 62.702) -> (-41.9115, 75.702)
  line L218 (-55.4115, 62.202) -> (-42.4115, 62.202)
  line L219 (-55.4115, 76.202) -> (-42.4115, 76.202)
  arc A216 (-55.9115, 62.702) -> (-55.4115, 62.202) centre (-55.4115, 62.702) ccw
  arc A217 (-55.4115, 76.202) -> (-55.9115, 75.702) centre (-55.4115, 75.702) ccw
  arc A218 (-42.4115, 62.202) -> (-41.9115, 62.702) centre (-42.4115, 62.702) ccw
  arc A219 (-41.9115, 75.702) -> (-42.4115, 76.202) centre (-42.4115, 75.702) ccw
  line L220 (-55.9115, 81.752) -> (-55.9115, 94.752)
  line L221 (-41.9115, 81.752) -> (-41.9115, 94.752)
  line L222 (-55.4115, 81.252) -> (-42.4115, 81.252)
  line L223 (-55.4115, 95.252) -> (-42.4115, 95.252)
  arc A220 (-55.9115, 81.752) -> (-55.4115, 81.252) centre (-55.4115, 81.752) ccw
  arc A221 (-55.4115, 95.252) -> (-55.9115, 94.752) centre (-55.4115, 94.752) ccw
  arc A222 (-42.4115, 81.252) -> (-41.9115, 81.752) centre (-42.4115, 81.752) ccw
  arc A223 (-41.9115, 94.752) -> (-42.4115, 95.252) centre (-42.4115, 94.752) ccw
  line L224 (-55.9115, 100.802) -> (-55.9115, 113.802)
  line L225 (-41.9115, 100.802) -> (-41.9115, 113.802)
  line L226 (-55.4115, 100.302) -> (-42.4115, 100.302)
  line L227 (-55.4115, 114.302) -> (-42.4115, 114.302)
  arc A224 (-55.9115, 100.802) -> (-55.4115, 100.302) centre (-55.4115, 100.802) ccw
  arc A225 (-55.4115, 114.302) -> (-55.9115, 113.802) centre (-55.4115, 113.802) ccw
  arc A226 (-42.4115, 100.302) -> (-41.9115, 100.802) centre (-42.4115, 100.802) ccw
  arc A227 (-41.9115, 113.802) -> (-42.4115, 114.302) centre (-42.4115, 113.802) ccw
  line L228 (-55.9115, 119.852) -> (-55.9115, 132.852)
  line L229 (-41.9115, 119.852) -> (-41.9115, 132.852)
  line L230 (-55.4115, 119.352) -> (-42.4115, 119.352)
  line L231 (-55.4115, 133.352) -> (-42.4115, 133.352)
  arc A228 (-55.9115, 119.852) -> (-55.4115, 119.352) centre (-55.4115, 119.852) ccw
  arc A229 (-55.4115, 133.352) -> (-55.9115, 132.852) centre (-55.4115, 132.852) ccw
  arc A230 (-42.4115, 119.352) -> (-41.9115, 119.852) centre (-42.4115, 119.852) ccw
  arc A231 (-41.9115, 132.852) -> (-42.4115, 133.352) centre (-42.4115, 132.852) ccw
  line L232 (-55.9115, 138.902) -> (-55.9115, 151.902)
  line L233 (-41.9115, 138.902) -> (-41.9115, 151.902)
  line L234 (-55.4115, 138.402) -> (-42.4115, 138.402)
  line L235 (-55.4115, 152.402) -> (-42.4115, 152.402)
  arc A232 (-55.9115, 138.902) -> (-55.4115, 138.402) centre (-55.4115, 138.902) ccw
  arc A233 (-55.4115, 152.402) -> (-55.9115, 151.902) centre (-55.4115, 151.902) ccw
  arc A234 (-42.4115, 138.402) -> (-41.9115, 138.902) centre (-42.4115, 138.902) ccw
  arc A235 (-41.9115, 151.902) -> (-42.4115, 152.402) centre (-42.4115, 151.902) ccw
  line L236 (-55.9115, 157.952) -> (-55.9115, 170.952)
  line L237 (-41.9115, 157.952) -> (-41.9115, 170.952)
  line L238 (-55.4115, 157.452) -> (-42.4115, 157.452)
  line L239 (-55.4115, 171.452) -> (-42.4115, 171.452)
  arc A236 (-55.9115, 157.952) -> (-55.4115, 157.452) centre (-55.4115, 157.952) ccw
  arc A237 (-55.4115, 171.452) -> (-55.9115, 170.952) centre (-55.4115, 170.952) ccw
  arc A238 (-42.4115, 157.452) -> (-41.9115, 157.952) centre (-42.4115, 157.952) ccw
  arc A239 (-41.9115, 170.952) -> (-42.4115, 171.452) centre (-42.4115, 170.952) ccw
  line L240 (-55.9115, 177.002) -> (-55.9115, 190.002)
  line L241 (-41.9115, 177.002) -> (-41.9115, 190.002)
  line L242 (-55.4115, 176.502) -> (-42.4115, 176.502)
  line L243 (-55.4115, 190.502) -> (-42.4115, 190.502)
  arc A240 (-55.9115, 177.002) -> (-55.4115, 176.502) centre (-55.4115, 177.002) ccw
  arc A241 (-55.4115, 190.502) -> (-55.9115, 190.002) centre (-55.4115, 190.002) ccw
  arc A242 (-42.4115, 176.502) -> (-41.9115, 177.002) centre (-42.4115, 177.002) ccw
  arc A243 (-41.9115, 190.002) -> (-42.4115, 190.502) centre (-42.4115, 190.002) ccw
  line L244 (-55.9115, 196.052) -> (-55.9115, 209.052)
  line L245 (-41.9115, 196.052) -> (-41.9115, 209.052)
  line L246 (-55.4115, 195.552) -> (-42.4115, 195.552)
  line L247 (-55.4115, 209.552) -> (-42.4115, 209.552)
  arc A244 (-55.9115, 196.052) -> (-55.4115, 195.552) centre (-55.4115, 196.052) ccw
  arc A245 (-55.4115, 209.552) -> (-55.9115, 209.052) centre (-55.4115, 209.052) ccw
  arc A246 (-42.4115, 195.552) -> (-41.9115, 196.052) centre (-42.4115, 196.052) ccw
  arc A247 (-41.9115, 209.052) -> (-42.4115, 209.552) centre (-42.4115, 209.052) ccw
  line L248 (-55.9115, 215.102) -> (-55.9115, 228.102)
  line L249 (-41.9115, 215.102) -> (-41.9115, 228.102)
  line L250 (-55.4115, 214.602) -> (-42.4115, 214.602)
  line L251 (-55.4115, 228.602) -> (-42.4115, 228.602)
  arc A248 (-55.9115, 215.102) -> (-55.4115, 214.602) centre (-55.4115, 215.102) ccw
  arc A249 (-55.4115, 228.602) -> (-55.9115, 228.102) centre (-55.4115, 228.102) ccw
  arc A250 (-42.4115, 214.602) -> (-41.9115, 215.102) centre (-42.4115, 215.102) ccw
  arc A251 (-41.9115, 228.102) -> (-42.4115, 228.602) centre (-42.4115, 228.102) ccw
  line L252 (-55.9115, 234.152) -> (-55.9115, 247.152)
  line L253 (-41.9115, 234.152) -> (-41.9115, 247.152)
  line L254 (-55.4115, 233.652) -> (-42.4115, 233.652)
  line L255 (-55.4115, 247.652) -> (-42.4115, 247.652)
  arc A252 (-55.9115, 234.152) -> (-55.4115, 233.652) centre (-55.4115, 234.152) ccw
  arc A253 (-55.4115, 247.652) -> (-55.9115, 247.152) centre (-55.4115, 247.152) ccw
  arc A254 (-42.4115, 233.652) -> (-41.9115, 234.152) centre (-42.4115, 234.152) ccw
  arc A255 (-41.9115, 247.152) -> (-42.4115, 247.652) centre (-42.4115, 247.152) ccw
  line L256 (-55.9115, 265.1082) -> (-55.9115, 278.1082)
  line L257 (-41.9115, 265.1082) -> (-41.9115, 278.1082)
  line L258 (-55.4115, 264.6082) -> (-42.4115, 264.6082)
  line L259 (-55.4115, 278.6082) -> (-42.4115, 278.6082)
  arc A256 (-55.9115, 265.1082) -> (-55.4115, 264.6082) centre (-55.4115, 265.1082) ccw
  arc A257 (-55.4115, 278.6082) -> (-55.9115, 278.1082) centre (-55.4115, 278.1082) ccw
  arc A258 (-42.4115, 264.6082) -> (-41.9115, 265.1082) centre (-42.4115, 265.1082) ccw
  arc A259 (-41.9115, 278.1082) -> (-42.4115, 278.6082) centre (-42.4115, 278.1082) ccw
  line L260 (-54.9115, 256.6702) -> (-54.9115, 262.6702)
  line L261 (-39.9115, 256.6702) -> (-39.9115, 262.6702)
  line L262 (-54.4115, 256.1702) -> (-40.4115, 256.1702)
  line L263 (-54.4115, 263.1702) -> (-40.4115, 263.1702)
  arc A260 (-54.9115, 256.6702) -> (-54.4115, 256.1702) centre (-54.4115, 256.6702) ccw
  arc A261 (-54.4115, 263.1702) -> (-54.9115, 262.6702) centre (-54.4115, 262.6702) ccw
  arc A262 (-40.4115, 256.1702) -> (-39.9115, 256.6702) centre (-40.4115, 256.6702) ccw
  arc A263 (-39.9115, 262.6702) -> (-40.4115, 263.1702) centre (-40.4115, 262.6702) ccw
  line L264 (-54.9115, 280.5462) -> (-54.9115, 286.5462)
  line L265 (-39.9115, 280.5462) -> (-39.9115, 286.5462)
  line L266 (-54.4115, 280.0462) -> (-40.4115, 280.0462)
  line L267 (-54.4115, 287.0462) -> (-40.4115, 287.0462)
  arc A264 (-54.9115, 280.5462) -> (-54.4115, 280.0462) centre (-54.4115, 280.5462) ccw
  arc A265 (-54.4115, 287.0462) -> (-54.9115, 286.5462) centre (-54.4115, 286.5462) ccw
  arc A266 (-40.4115, 280.0462) -> (-39.9115, 280.5462) centre (-40.4115, 280.5462) ccw
  arc A267 (-39.9115, 286.5462) -> (-40.4115, 287.0462) centre (-40.4115, 286.5462) ccw
  line L268 (-36.8615, 22.2207) -> (-36.8615, 35.2207)
  line L269 (-22.8615, 22.2207) -> (-22.8615, 35.2207)
  line L270 (-36.3615, 21.7207) -> (-23.3615, 21.7207)
  line L271 (-36.3615, 35.7207) -> (-23.3615, 35.7207)
  arc A268 (-36.8615, 22.2207) -> (-36.3615, 21.7207) centre (-36.3615, 22.2207) ccw
  arc A269 (-36.3615, 35.7207) -> (-36.8615, 35.2207) centre (-36.3615, 35.2207) ccw
  arc A270 (-23.3615, 21.7207) -> (-22.8615, 22.2207) centre (-23.3615, 22.2207) ccw
  arc A271 (-22.8615, 35.2207) -> (-23.3615, 35.7207) centre (-23.3615, 35.2207) ccw
  line L272 (-35.8615, 13.7827) -> (-35.8615, 19.7827)
  line L273 (-20.8615, 13.7827) -> (-20.8615, 19.7827)
  line L274 (-35.3615, 13.2827) -> (-21.3615, 13.2827)
  line L275 (-35.3615, 20.2827) -> (-21.3615, 20.2827)
  arc A272 (-35.8615, 13.7827) -> (-35.3615, 13.2827) centre (-35.3615, 13.7827) ccw
  arc A273 (-35.3615, 20.2827) -> (-35.8615, 19.7827) centre (-35.3615, 19.7827) ccw
  arc A274 (-21.3615, 13.2827) -> (-20.8615, 13.7827) centre (-21.3615, 13.7827) ccw
  arc A275 (-20.8615, 19.7827) -> (-21.3615, 20.2827) centre (-21.3615, 19.7827) ccw
  line L276 (-35.8615, 37.6587) -> (-35.8615, 43.6587)
  line L277 (-20.8615, 37.6587) -> (-20.8615, 43.6587)
  line L278 (-35.3615, 37.1587) -> (-21.3615, 37.1587)
  line L279 (-35.3615, 44.1587) -> (-21.3615, 44.1587)
  arc A276 (-35.8615, 37.6587) -> (-35.3615, 37.1587) centre (-35.3615, 37.6587) ccw
  arc A277 (-35.3615, 44.1587) -> (-35.8615, 43.6587) centre (-35.3615, 43.6587) ccw
  arc A278 (-21.3615, 37.1587) -> (-20.8615, 37.6587) centre (-21.3615, 37.6587) ccw
  arc A279 (-20.8615, 43.6587) -> (-21.3615, 44.1587) centre (-21.3615, 43.6587) ccw
  line L280 (-36.8615, 53.177) -> (-36.8615, 66.177)
  line L281 (-22.8615, 53.177) -> (-22.8615, 66.177)
  line L282 (-36.3615, 52.677) -> (-23.3615, 52.677)
  line L283 (-36.3615, 66.677) -> (-23.3615, 66.677)
  arc A280 (-36.8615, 53.177) -> (-36.3615, 52.677) centre (-36.3615, 53.177) ccw
  arc A281 (-36.3615, 66.677) -> (-36.8615, 66.177) centre (-36.3615, 66.177) ccw
  arc A282 (-23.3615, 52.677) -> (-22.8615, 53.177) centre (-23.3615, 53.177) ccw
  arc A283 (-22.8615, 66.177) -> (-23.3615, 66.677) centre (-23.3615, 66.177) ccw
  line L284 (-36.8615, 72.227) -> (-36.8615, 85.227)
  line L285 (-22.8615, 72.227) -> (-22.8615, 85.227)
  line L286 (-36.3615, 71.727) -> (-23.3615, 71.727)
  line L287 (-36.3615, 85.727) -> (-23.3615, 85.727)
  arc A284 (-36.8615, 72.227) -> (-36.3615, 71.727) centre (-36.3615, 72.227) ccw
  arc A285 (-36.3615, 85.727) -> (-36.8615, 85.227) centre (-36.3615, 85.227) ccw
  arc A286 (-23.3615, 71.727) -> (-22.8615, 72.227) centre (-23.3615, 72.227) ccw
  arc A287 (-22.8615, 85.227) -> (-23.3615, 85.727) centre (-23.3615, 85.227) ccw
  line L288 (-36.8615, 91.277) -> (-36.8615, 104.277)
  line L289 (-22.8615, 91.277) -> (-22.8615, 104.277)
  line L290 (-36.3615, 90.777) -> (-23.3615, 90.777)
  line L291 (-36.3615, 104.777) -> (-23.3615, 104.777)
  arc A288 (-36.8615, 91.277) -> (-36.3615, 90.777) centre (-36.3615, 91.277) ccw
  arc A289 (-36.3615, 104.777) -> (-36.8615, 104.277) centre (-36.3615, 104.277) ccw
  arc A290 (-23.3615, 90.777) -> (-22.8615, 91.277) centre (-23.3615, 91.277) ccw
  arc A291 (-22.8615, 104.277) -> (-23.3615, 104.777) centre (-23.3615, 104.277) ccw
  line L292 (-36.8615, 110.327) -> (-36.8615, 123.327)
  line L293 (-22.8615, 110.327) -> (-22.8615, 123.327)
  line L294 (-36.3615, 109.827) -> (-23.3615, 109.827)
  line L295 (-36.3615, 123.827) -> (-23.3615, 123.827)
  arc A292 (-36.8615, 110.327) -> (-36.3615, 109.827) centre (-36.3615, 110.327) ccw
  arc A293 (-36.3615, 123.827) -> (-36.8615, 123.327) centre (-36.3615, 123.327) ccw
  arc A294 (-23.3615, 109.827) -> (-22.8615, 110.327) centre (-23.3615, 110.327) ccw
  arc A295 (-22.8615, 123.327) -> (-23.3615, 123.827) centre (-23.3615, 123.327) ccw
  line L296 (-36.8615, 129.377) -> (-36.8615, 142.377)
  line L297 (-22.8615, 129.377) -> (-22.8615, 142.377)
  line L298 (-36.3615, 128.877) -> (-23.3615, 128.877)
  line L299 (-36.3615, 142.877) -> (-23.3615, 142.877)
  arc A296 (-36.8615, 129.377) -> (-36.3615, 128.877) centre (-36.3615, 129.377) ccw
  arc A297 (-36.3615, 142.877) -> (-36.8615, 142.377) centre (-36.3615, 142.377) ccw
  arc A298 (-23.3615, 128.877) -> (-22.8615, 129.377) centre (-23.3615, 129.377) ccw
  arc A299 (-22.8615, 142.377) -> (-23.3615, 142.877) centre (-23.3615, 142.377) ccw
  line L300 (-36.8615, 148.427) -> (-36.8615, 161.427)
  line L301 (-22.8615, 148.427) -> (-22.8615, 161.427)
  line L302 (-36.3615, 147.927) -> (-23.3615, 147.927)
  line L303 (-36.3615, 161.927) -> (-23.3615, 161.927)
  arc A300 (-36.8615, 148.427) -> (-36.3615, 147.927) centre (-36.3615, 148.427) ccw
  arc A301 (-36.3615, 161.927) -> (-36.8615, 161.427) centre (-36.3615, 161.427) ccw
  arc A302 (-23.3615, 147.927) -> (-22.8615, 148.427) centre (-23.3615, 148.427) ccw
  arc A303 (-22.8615, 161.427) -> (-23.3615, 161.927) centre (-23.3615, 161.427) ccw
  line L304 (-36.8615, 167.477) -> (-36.8615, 180.477)
  line L305 (-22.8615, 167.477) -> (-22.8615, 180.477)
  line L306 (-36.3615, 166.977) -> (-23.3615, 166.977)
  line L307 (-36.3615, 180.977) -> (-23.3615, 180.977)
  arc A304 (-36.8615, 167.477) -> (-36.3615, 166.977) centre (-36.3615, 167.477) ccw
  arc A305 (-36.3615, 180.977) -> (-36.8615, 180.477) centre (-36.3615, 180.477) ccw
  arc A306 (-23.3615, 166.977) -> (-22.8615, 167.477) centre (-23.3615, 167.477) ccw